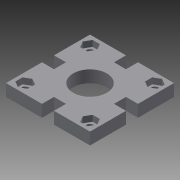
# Autodesk Inventor part: crossCenter
Saved by Autodesk Inventor 2015 (Build 190159000, 159)
## iProperties
Created: 2016-10-14
Part Number: crossCenter
Material: Generic
Document SubType Name: Modeling
Designer: Bardo91
Density: 1 g/cm^3
Appearance: Default
Author: Bardo91
Autodesk Inventor part; units mm, degrees
ref_plane "YZ Plane" through (0, 0, 0) normal (1, 0, 0) x (0, 1, 0)
ref_plane "XZ Plane" through (0, 0, 0) normal (0, 1, 0) x (-1, 0, 0)
ref_plane "XY Plane" through (0, 0, 0) normal (0, 0, 1) x (1, 0, 0)
sketch "Sketch1" plane through (0, 0, 0) normal (0, 0, 1) x (1, 0, 0)
  line L0 (0, 0) -> (-5, 0)
  line L1 (-5, 0) -> (-5, 2.5)
  line L2 (-5, 2.5) -> (-10, 2.5)
  line L3 (-10, 2.5) -> (-10, 7.5)
  line L4 (-10, 7.5) -> (-5, 7.5)
  line L5 (-5, 7.5) -> (-5, 12.5)
  line L6 (-5, 12.5) -> (0, 12.5)
  line L7 (-5, 0) -> (-5, -2.5)
  line L8 (-5, -2.5) -> (-10, -2.5)
  line L9 (-10, -2.5) -> (-10, -7.5)
  line L10 (-10, -7.5) -> (-5, -7.5)
  line L11 (-5, -7.5) -> (-5, -12.5)
  line L12 (-5, -12.5) -> (0, -12.5)
  line L13 (0, 12.5) -> (0, 17.5)
  line L14 (0, 17.5) -> (5, 17.5)
  line L15 (5, 17.5) -> (5, 12.5)
  line L16 (5, 12.5) -> (10, 12.5)
  line L17 (10, 12.5) -> (10, 17.5)
  line L18 (10, 17.5) -> (15, 17.5)
  line L19 (15, 17.5) -> (15, 12.5)
  line L20 (15, 12.5) -> (20, 12.5)
  line L21 (20, 12.5) -> (20, 7.5)
  line L22 (20, 7.5) -> (25, 7.5)
  line L23 (25, 7.5) -> (25, 2.5)
  line L24 (25, 2.5) -> (20, 2.5)
  line L25 (20, 2.5) -> (20, -2.5)
  line L26 (20, -2.5) -> (25, -2.5)
  line L27 (25, -2.5) -> (25, -7.5)
  line L28 (25, -7.5) -> (20, -7.5)
  line L29 (20, -7.5) -> (20, -12.5)
  line L30 (20, -12.5) -> (15, -12.5)
  line L31 (15, -12.5) -> (15, -17.5)
  line L32 (15, -17.5) -> (10, -17.5)
  line L33 (10, -17.5) -> (10, -12.5)
  line L34 (10, -12.5) -> (5, -12.5)
  line L35 (5, -12.5) -> (5, -17.5)
  line L36 (5, -17.5) -> (0, -17.5)
  line L37 (0, -17.5) -> (0, -12.5)
  line L38 (0, 17.5) -> (-10, 17.5)
  line L39 (-10, 17.5) -> (-10, 7.5)
  line L40 (15, 17.5) -> (25, 17.5)
  line L41 (25, 17.5) -> (25, 7.5)
  line L42 (25, -7.5) -> (25, -17.5)
  line L43 (25, -17.5) -> (15, -17.5)
  line L44 (0, -17.5) -> (-10, -17.5)
  line L45 (-10, -7.5) -> (-10, -17.5)
  dimension "d0" = 5
  dimension "d1" = 2.5
  dimension "d2" = 5
  dimension "d3" = 5
  dimension "d4" = 5
  dimension "d5" = 5
  dimension "d6" = 5
  dimension "d7" = 2.5
  dimension "d8" = 5
  dimension "d9" = 5
  dimension "d10" = 5
  dimension "d11" = 5
  dimension "d12" = 5
  dimension "d13" = 5
  dimension "d14" = 5
  dimension "d15" = 5
  dimension "d16" = 5
  dimension "d17" = 5
  dimension "d18" = 5
  dimension "d19" = 5
  dimension "d20" = 5
  dimension "d21" = 5
  dimension "d22" = 5
  dimension "d23" = 5
  dimension "d24" = 5
  dimension "d25" = 5
  dimension "d26" = 5
  dimension "d27" = 5
  dimension "d28" = 5
  dimension "d29" = 5
  dimension "d30" = 5
  dimension "d31" = 5
  dimension "d32" = 5
  constraints: 92 end point, 24 point on line, 21 perpendicular, 3 vertical, 1 horizontal
  measures "d0" distance of L0.start L0.end
  measures "d1" distance of L0.end L1.end
  measures "d2" distance of L1.end L2.end
  measures "d3" distance of L2.end L3.end
  measures "d4" distance of L3.end L4.end
  measures "d5" distance of L4.end L5.end
  measures "d6" distance of L5.end L6.end
  measures "d7" distance of L0.end L7.end
  measures "d8" distance of L8.end L9.end
  measures "d9" distance of L10.end L11.end
  measures "d10" distance of L11.end L12.end
  measures "d11" distance of L6.end L13.end
  measures "d12" distance of L13.end L14.end
  measures "d13" distance of L14.end L15.end
  measures "d14" distance of L15.end L16.end
  measures "d15" distance of L17.end L18.end
  measures "d16" distance of L18.end L19.end
  measures "d17" distance of L19.end L20.end
  measures "d18" distance of L20.end L21.end
  measures "d19" distance of L21.end L22.end
  measures "d20" distance of L22.end L23.end
  measures "d21" distance of L23.end L24.end
  measures "d22" distance of L24.end L25.end
  measures "d23" distance of L26.end L27.end
  measures "d24" distance of L27.end L28.end
  measures "d25" distance of L28.end L29.end
  measures "d26" distance of L29.end L30.end
  measures "d27" distance of L30.end L31.end
  measures "d28" distance of L31.end L32.end
  measures "d29" distance of L32.end L33.end
  measures "d30" distance of L33.end L34.end
  measures "d31" distance of L34.end L35.end
  measures "d32" distance of L35.end L36.end
extrude "Extrusion1" add sketch "Sketch1" along normal blind 5
sketch "Sketch4" plane through (0, 0, 5) normal (0, 0, 1) x (1, 0, 0)
  line L0 (-10, 17.5) -> (-10, 13.5)
  line L1 (-10, 17.5) -> (-10, 2.5) projected
  line L2 (-10, 13.5) -> (-6, 13.5)
  circle A0 centre (-6, 13.5) radius 1.75
  point P0 (0, 0)
  dimension "d54" = 4
  dimension "d55" = 4
  dimension "d56" = 3.5
  constraints: 4 end point, 1 centre point, 1 coincident, 1 perpendicular, 1 point on line
  measures "d54" distance of L0.start L0.end
  measures "d55" distance of L0.end L2.end
  measures "d56" diameter of A0
extrude "Extrusion4" cut sketch "Sketch4" against normal blind 10
sketch "Sketch5" plane through (0, 0, 5) normal (0, 0, 1) x (1, 0, 0)
  circle A0 centre (-6, 13.5) radius 1.75 projected
  line L0 (-6, 13.5) -> (-3, 13.5)
  line L1 (-3, 13.5) -> (-4.5, 16.0981)
  line L2 (-4.5, 16.0981) -> (-6, 13.5)
  point P0 (0, 0)
  dimension "d59" = 3
  dimension "d60" = 3
  dimension "d61" = 60
  constraints: 6 end point, 1 horizontal
  measures "d59" distance of L0.start L0.end
  measures "d60" distance of L0.end L1.end
  measures "d61" angle of L1 L0
extrude "Extrusion5" cut sketch "Sketch5" against normal blind 2.5 contours L0 L2 A0 | A0 L2 L1 L0 picked at (-4.9952, 14.0801)
pattern_circular "Circular Pattern2" count 6 over 360 about axis through (-6, 13.5, 5) along (0, 0, -1) of "Extrusion5"
sketch "Sketch6" plane through (0, 0, 5) normal (0, 0, 1) x (1, 0, 0)
  line L0 (-5, -2.5) -> (-5, 2.5) projected
  line L1 (-5, 0) -> (20, 0)
  line L2 (20, 2.5) -> (20, -2.5) projected
  line L3 (5, 12.5) -> (10, 12.5) projected
  line L4 (7.5, 12.5) -> (7.5, 0)
  circle A0 centre (7.5, 0) radius 7
  point P0 (0, 0)
  dimension "d70" = 14
  constraints: 4 end point, 4 midpoint, 1 centre point, 1 coincident
  measures "d70" diameter of A0
extrude "Extrusion6" cut sketch "Sketch6" against normal through all
pattern_circular "Circular Pattern4" count 4 over 360 about axis through (7.5, 0, 5) along (0, 0, -1) of "Extrusion5", "Circular Pattern2", "Extrusion4"
body "Solid1"
